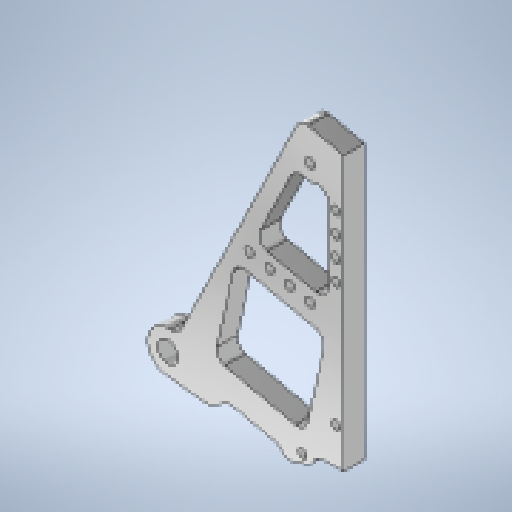
# Autodesk Inventor part: Uprights
Saved by Autodesk Inventor 2023.2 (Build 272271000, 271)
## iProperties
Created: 2024-02-11
Part Number: Uprights
Material: Aluminum 6061
Document SubType Name: Modeling
Designer: Nathan Cai
Density: 2.7 g/cm^3
Appearance: Aluminum - Flat
Mass: 31.1951 g
Surface Area: 70.3798 cm^2
Volume: 11.5537 cm^3
Author: Nathan Cai
Autodesk Inventor part; units mm, degrees
ref_plane "YZ Plane" through (0, 0, 0) normal (1, 0, 0) x (0, 1, 0)
ref_plane "XZ Plane" through (0, 0, 0) normal (0, 1, 0) x (-1, 0, 0)
ref_plane "XY Plane" through (0, 0, 0) normal (0, 0, 1) x (1, 0, 0)
sketch "Sketch1" plane through (0, 0, 0) normal (0, 0, 1) x (1, 0, 0)
  line L0 (0, 0) -> (0, 136.525)
  line L1 (-11.7886, 12.2907) -> (-39.6863, 18.4755)
  line L2 (-39.6863, 18.4755) -> (-33.3297, 47.1481)
  line L3 (-33.3297, 47.1481) -> (-5.432, 40.9633)
  line L4 (-5.432, 40.9633) -> (-11.7886, 12.2907)
  line L5 (-39.6863, 18.4755) -> (-5.432, 40.9633) construction
  line L6 (-33.3297, 47.1481) -> (-11.7886, 12.2907) construction
  circle A0 centre (-53.975, 12.7) radius 3.175
  circle A1 centre (-53.975, 12.7) radius 6.35
  line L7 (0, 0) -> (-54.712, 6.3929)
  line L8 (-59.6703, 15.5082) -> (0, 136.525)
  line L9 (-27.1302, 45.7737) -> (-37.4529, 28.5497)
  line L10 (-11.6315, 42.3377) -> (-9.5552, 22.3649)
  line L11 (-19.3809, 44.0557) -> (-25.7374, 15.3831) construction
  line L12 (0, 92.075) -> (-19.7574, 96.4551)
  line L13 (-35.3766, 8.5768) -> (-19.8779, 5.1408)
  line L14 (-19.8779, 5.1408) -> (-21.2523, -1.0586)
  line L15 (-21.2523, -1.0586) -> (-36.751, 2.3773)
  line L16 (-36.751, 2.3773) -> (-35.3766, 8.5768)
  line L17 (-35.3766, 8.5768) -> (-41.27, 4.8223)
  line L18 (-19.8779, 5.1408) -> (-17.9381, 2.096)
  line L19 (-5.432, 40.9633) -> (-33.3297, 47.1481)
  line L20 (-33.3297, 47.1481) -> (-32.2475, 52.0296)
  line L21 (-32.2475, 52.0296) -> (-4.3498, 45.8448)
  line L22 (-4.3498, 45.8448) -> (-5.432, 40.9633)
  line L23 (-53.2878, 15.7997) -> (-53.975, 12.7) construction
  line L24 (-53.975, 12.7) -> (-57.0747, 13.3872) construction
  line L25 (-27.6272, 6.8588) -> (-34.4992, -24.1386) construction
  line L26 (-31.8676, 50.076) -> (-5.5198, 44.2349)
  line L27 (-5.5198, 44.2349) -> (-4.489, 48.8845)
  line L28 (-4.489, 48.8845) -> (-30.8368, 54.7256)
  line L29 (-30.8368, 54.7256) -> (-31.8676, 50.076)
  line L30 (-31.3522, 52.4008) -> (-5.0044, 46.5597) construction
  circle A2 centre (-29.0274, 51.8854) radius 1.4732
  circle A3 centre (-22.8279, 50.5111) radius 1.4732
  circle A4 centre (-16.6284, 49.1367) radius 1.4732
  circle A5 centre (-10.4289, 47.7623) radius 1.4732
  circle A6 centre (-10.3614, 84.7398) radius 1.4732
  line L31 (-53.975, 12.7) -> (-13.3751, 95.0402)
  line L32 (-32.2923, 56.6744) -> (0, 49.5153)
  circle A7 centre (-10.3614, 84.7398) radius 4.7625
  line L33 (-4.7625, 50.5712) -> (-4.7625, 93.1308)
  line L34 (-27.5056, 55.6132) -> (-14.3936, 82.2055)
  line L35 (-5.6003, 84.6261) -> (-4.7625, 84.4403)
  circle A8 centre (-12.7, 6.35) radius 1.4224
  line L36 (-9.525, 4.7625) -> (-17.9381, 2.096)
  line L37 (-9.525, 7.9375) -> (-9.525, 4.7625)
  line L38 (-9.525, 7.9375) -> (0, 7.9375)
  line L39 (0, 13.4938) -> (-4.7625, 13.4937) construction
  line L40 (-4.7625, 13.4937) -> (-4.7625, 24.6063) construction
  line L41 (-4.7625, 24.6063) -> (0, 24.6063) construction
  line L42 (0, 24.6063) -> (0, 13.4938) construction
  line L43 (-4.7625, 19.05) -> (0, 19.05) construction
  circle A9 centre (-2.3812, 19.05) radius 1.4224
  line L44 (-4.7625, 57.15) -> (0, 57.15) construction
  circle A10 centre (-2.3813, 57.15) radius 1.4224
  circle A11 centre (-2.3813, 63.5) radius 1.4224
  circle A12 centre (-2.3813, 69.85) radius 1.4224
  circle A13 centre (-2.3813, 76.2) radius 1.4224
  line L45 (-34.4992, -24.1386) -> (-14.5705, 65.7539) construction
  line L46 (-14.5705, 65.7539) -> (-17.3193, 53.3549) construction
  line L47 (-17.3193, 53.3549) -> (-11.1198, 51.9805) construction
  line L48 (-11.1198, 51.9805) -> (-8.371, 64.3795) construction
  line L49 (-8.371, 64.3795) -> (-14.5705, 65.7539) construction
  line L50 (-14.2195, 52.6677) -> (-11.4708, 65.0667) construction
  line L51 (-15.9449, 59.5544) -> (-9.7454, 58.18) construction
  line L52 (-17.3193, 53.3549) -> (-9.7454, 58.18) construction
  line L53 (-14.5705, 65.7539) -> (-9.7454, 58.18) construction
  circle A14 centre (-13.5323, 55.7675) radius 1.4224
  circle A15 centre (-12.1579, 61.967) radius 1.4224
  line L54 (-14.2195, 52.6677) -> (-12.1579, 61.967) construction
  line L55 (-11.1198, 51.9805) -> (-9.0582, 61.2798)
  line L56 (-15.2577, 62.6542) -> (-17.3193, 53.3549)
  arc A16 (-17.3193, 53.3549) -> (-11.1198, 51.9805) centre (-14.2195, 52.6677) ccw construction
  arc A17 (-9.0582, 61.2798) -> (-15.2577, 62.6542) centre (-12.1579, 61.967) ccw
  point P0 (-22.5591, 29.7194)
  point P1 (-20.4869, 2.3938)
  point P2 (-36.3367, 4.2458)
  point P3 (-51.1668, 18.3953)
  point P4 (-4.7625, 7.9375)
  point P5 (-22.5591, 29.7194)
  point P6 (-13.1887, 57.3173)
  dimension "d13" = 136.525
  dimension "d14" = 29.3687
  dimension "d15" = 28.575
  dimension "d16" = 12.5
  dimension "d17" = 6.35
  dimension "d19" = 53.975
  dimension "d22" = 12.7
  dimension "d23" = 7.9375
  dimension "d24" = 19.05
  dimension "d26" = 102.5
  dimension "d29" = 6.35
  dimension "d31" = 7.9375
  dimension "d34" = 5
  dimension "d35" = 26.9875
  dimension "d38" = 31.75
  dimension "d40" = 26.9875
  dimension "d41" = 4.7625
  dimension "d42" = 2.9464
  dimension "d43" = 2.3813
  dimension "d46" = 6.35
  dimension "d51" = 2.9464
  dimension "d52" = 79.7719
  dimension "d53" = 6.35
  dimension "d54" = 9.525
  dimension "d55" = 4.7625
  dimension "d56" = 4.7625
  dimension "d60" = 12.7
  dimension "d61" = 3.175
  dimension "d66" = 2.8448
  dimension "d67" = 12.7
  dimension "d72" = 8.7312
  dimension "d75" = 34.925
  dimension "d80" = 92.075
  dimension "d81" = 6.35
  dimension "d82" = 7.9375
  dimension "d83" = 3.175
  dimension "d84" = 9.525
  dimension "d85" = 4.7625
  dimension "d86" = 11.1125
  dimension "d87" = 2.8448
  dimension "d88" = 19.05
  dimension "d89" = 2.8448
  dimension "d90" = 38.1
  dimension "d93" = 6.35
  dimension "d98" = 92.075
  dimension "d99" = 12.7
  dimension "d100" = 6.35
  dimension "d101" = 2.8448
  dimension "d102" = 2.8448
  constraints: 116 end point, 24 point on line, 20 parallel, 19 midpoint, 18 centre point, 11 perpendicular, 10 point on circle, 9 coincident, 7 tangent, 3 vertical, 2 collinear, 1 horizontal, 17 other
  measures "d13" distance of L0.start L0.end
  measures "d14" distance of L1.end L2.end
  measures "d15" distance between parallel lines of L4 L2
  measures "d16" angle of L0 L4
  measures "d17" diameter of A0
  measures "d19" distance from line of L0 A0.centre
  measures "d22" diameter of A1
  measures "d23" distance from line of L9.start L11
  measures "d24" distance from line of L9.end L3
  measures "d26" angle of L0 L12
  measures "d29" distance of L13.end L14.end
  measures "d31" distance between parallel lines of L14 L11
  measures "d34" distance of L2.end L20.end
  measures "d35" distance between parallel lines of L11 L23
  measures "d38" distance of L25.start L25.end
  measures "d40" distance between parallel lines of L27 L29
  measures "d41" distance between parallel lines of L26 L28
  measures "d42" diameter of A2
  measures "d43" distance from line of L29 A2.centre
  measures "d46" distance of A2.centre A3.centre
  measures "d51" diameter of A6
  measures "d52" distance from line of L13 A6.centre
  measures "d53" distance between parallel lines of L32 L26
  measures "d54" diameter of A7
  measures "d55" distance between parallel lines of L0 L33
  measures "d56" distance between parallel lines of L31 L34
  measures "d60" vertical distance of A0.centre L0.start
  measures "d61" distance between parallel lines of L3 L26
  measures "d66" diameter of A8
  measures "d67" distance from line of L0 A8.centre
  measures "d72" distance between parallel lines of L1 L13
  measures "d75" vertical distance of point (0, 49.515) point (-4.763, 84.44)
  measures "d80" distance of L0.start point (0, 92.075)
  measures "d81" vertical distance of L0.start A8.centre
  measures "d82" distance from line of L0.start L38
  measures "d83" vertical distance of point (-4.763, 7.937) L36.start
  measures "d84" distance between parallel lines of L0 L37
  measures "d85" distance of L40.end L41.end
  measures "d86" distance between parallel lines of L39 L41
  measures "d87" diameter of A9
  measures "d88" distance from line of point (0, 0) L43
  measures "d89" diameter of A10
  measures "d90" distance between parallel lines of L43 L44
  measures "d93" distance of A10.centre A11.centre
  measures "d98" distance of L25.end L45.end
  measures "d99" distance of L45.end L46.end
  measures "d100" distance of L47.end L46.end
  measures "d101" diameter of A14
  measures "d102" diameter of A15
extrude "Extrusion1" add sketch "Sketch1" along normal blind 6.35 contours L38 L37 L36 L18 L13 L17 L7 A1 L31 L32 L0 | L32 L33 L12 L0 | L33 L35 A7 L34 L32 L31 L12 | A7 | A1 | L3 L20 L21 L29 L26 L27 L22 | L27 L26 L29 L21 A2 A3 A4 A5 | L21 A5 A4 A3 A2 L29 L28 L27
fillet "Fillet1" radius 3.175 17 edges at (-39.6863, 18.4755, 3.175) (-11.7886, 12.2907, 3.175) (-51.1668, 18.3953, 3.175) (-19.8779, 5.1408, 3.175) (-35.3766, 8.5768, 3.175) (-41.27, 4.8223, 3.175) (-13.3751, 95.0402, 3.175) (-14.3936, 82.2055, 3.175) (-5.6003, 84.6261, 3.175) (-4.7625, 84.4403, 3.175) (-27.5056, 55.6132, 3.175) (-4.7625, 50.5712, 3.175) (-33.3297, 47.1481, 3.175) (-5.432, 40.9633, 3.175) (-17.9381, 2.096, 3.175) (-9.525, 7.9375, 3.175) (-9.525, 4.7625, 3.175)
equation "\"d56\" = d55"
body "Solid1"
